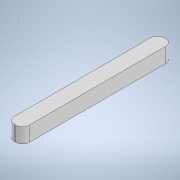
# Autodesk Inventor part: Maybe CIM Key
Saved by Autodesk Inventor 2020 (Build 240168000, 168)
## iProperties
Created: 2020-02-02
Part Number: Maybe CIM Key
Material: Generic
Document SubType Name: Modeling
Designer: aidan
Density: 1 g/cm^3
Appearance: Default
Author: aidan
Autodesk Inventor part; units mm, degrees
ref_plane "YZ Plane" through (0, 0, 0) normal (1, 0, 0) x (0, 1, 0)
ref_plane "XZ Plane" through (0, 0, 0) normal (0, 1, 0) x (-1, 0, 0)
ref_plane "XY Plane" through (0, 0, 0) normal (0, 0, 1) x (1, 0, 0)
sketch "Sketch1" plane through (0, 0, 0) normal (0, 0, 1) x (1, 0, 0)
  line L0 (-0.7792, 0.974) -> (1.2208, 0.974)
  line L1 (1.2208, 0.974) -> (1.2208, -1.026)
  line L2 (1.2208, -1.026) -> (-0.7792, -1.026)
  line L3 (-0.7792, -1.026) -> (-0.7792, 0.974)
  point P0 (0, 0)
  dimension "d0" = 2
  constraints: 8 end point, 2 parallel, 2 perpendicular, 1 horizontal
  measures "d0" distance of L0.start L0.end
extrude "Extrusion1" add sketch "Sketch1" along normal blind 20
fillet "Fillet1" radius 0.889 4 edges at (-0.7792, -0.026, 20) (1.2208, -0.026, 20) (1.2208, -0.026, 0) (-0.7792, -0.026, 0)
body "Solid1"
